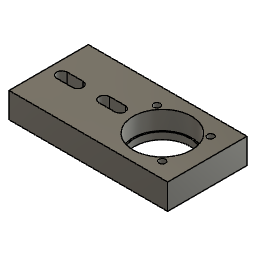
BeltTensionerBlock v21 (Autodesk Fusion 360 archive; units mm, degrees)
design "BeltTensionerBlock" references "tormach 770mx"
Autodesk Fusion 360 part; units mm, degrees
sketch "Sketch1" plane through (0, 0, 0) normal (0, 1, 0) x (1, 0, 0)
  line L0 (0, 0) -> (60, 0)
  line L1 (60, 0) -> (60, -30)
  line L2 (60, -30) -> (0, -30)
  line L3 (0, -30) -> (0, 0)
  line L4 (0, -15) -> (60, -15) construction
  line L5 (8, 0) -> (8, -30) construction
  line L6 (24, 0) -> (24, -30) construction
  line L7 (11, -13) -> (5, -13)
  arc A0 (5, -13) -> (5, -17) centre (5, -15) ccw
  line L8 (5, -17) -> (11, -17)
  arc A1 (11, -17) -> (11, -13) centre (11, -15) ccw
  line L9 (11, -15) -> (5, -15) construction
  line L10 (21, -17) -> (27, -17)
  arc A2 (27, -17) -> (27, -13) centre (27, -15) ccw
  line L11 (27, -13) -> (21, -13)
  arc A3 (21, -13) -> (21, -17) centre (21, -15) ccw
  line L12 (21, -15) -> (27, -15) construction
  line L13 (43, 0) -> (43, -30) construction
  point P0 (11, -15)
  point P1 (5, -15)
  point P2 (21, -15)
  point P3 (27, -15)
  dimension "d1" = 60
  dimension "d2" = 30
  dimension "d3" = 8
  dimension "d4" = 16
  dimension "d5" = 3
  dimension "d6" = 3
  dimension "d7" = 3
  dimension "d8" = 3
  dimension "d9" = 4
  dimension "d10" = 4
  dimension "d13" = 43
  constraint horizontal L0
  constraint vertical L1
  constraint horizontal L2
  constraint vertical L3
  constraint coincident L0.start L3.end
  constraint midpoint L3 L4.start
  constraint midpoint L1 L4.end
  constraint coincident L0 L5.start
  constraint coincident L2 L5.end
  constraint perpendicular L2 L5
  constraint coincident L0 L6.start
  constraint coincident L2 L6.end
  constraint perpendicular L2 L6
  constraint coincident L4 P0
  constraint coincident L4 P1
  constraint coincident L4 P2
  constraint coincident L4 P3
  constraint tangent L7 A0
  constraint tangent A0 L8
  constraint parallel L7 L8
  constraint tangent L8 A1
  constraint tangent L7 A1
  constraint coincident P1 A0.centre
  constraint perpendicular L5 L9
  constraint coincident P0 A1.centre
  constraint tangent L10 A2
  constraint tangent A2 L11
  constraint parallel L10 L11
  constraint tangent L11 A3
  constraint tangent L10 A3
  constraint coincident P3 A2.centre
  constraint perpendicular L6 L12
  constraint coincident P2 A3.centre
  constraint coincident L0 L13.start
  constraint coincident L2 L13.end
  constraint perpendicular L2 L13
  measures "d1" distance of L0.start L0.end
  measures "d2" distance of L0.start L2.end
  measures "d3" distance of L3 L5
  measures "d4" distance of L5 L6
  measures "d5" distance of L5 P1
  measures "d6" distance of L5 P0
  measures "d7" distance of L6 P2
  measures "d8" distance of L6 P3
  measures "d9" diameter of A0
  measures "d10" diameter of A2
  measures "d13" distance of L3 L13
extrude "Extrude1" add sketch "Sketch1" along normal blind 9.6
sketch "Sketch2" plane through (0, 9.6, 0) normal (0, 1, 0) x (-1, 0, 0)
  arc A0 (-21, 13) -> (-21, 17) centre (-21, 15) ccw
  line L0 (-21, 13) -> (-27, 13)
  arc A1 (-27, 17) -> (-27, 13) centre (-27, 15) ccw
  line L1 (-27, 17) -> (-21, 17)
  arc A2 (-11, 17) -> (-11, 13) centre (-11, 15) ccw
  line L2 (-11, 17) -> (-5, 17)
  arc A3 (-5, 13) -> (-5, 17) centre (-5, 15) ccw
  line L3 (-5, 13) -> (-11, 13)
  line L4 (0, 30) -> (-60, 30)
  line L5 (-60, 30) -> (-60, 0)
  line L6 (-60, 0) -> (0, 0)
  line L7 (0, 0) -> (0, 30)
  circle A4 centre (-43, 15) radius 11.05
  circle A5 centre (-43, 15) radius 10.55
  dimension "d15" = 22.1
  dimension "d16" = 21.1
  constraint concentric A4 A5
  measures "d15" diameter of A4
  measures "d16" diameter of A5
extrude "Extrude2" cut sketch "Sketch2" against normal blind 7 contours A4
extrude "Extrude3" cut 1 faces at (40.0944, 9.6, 14.0673) along direction (0, 1, 0) through all and the other way through all
sketch "Sketch3" plane through (0, 9.6, 0) normal (0, 1, 0) x (-1, 0, 0)
  line L0 (0, 30) -> (-60, 30)
  line L1 (-60, 30) -> (-60, 0)
  line L2 (-60, 0) -> (0, 0)
  line L3 (0, 0) -> (0, 30)
  arc A0 (-21, 13) -> (-21, 17) centre (-21, 15) ccw
  line L4 (-21, 13) -> (-27, 13)
  arc A1 (-27, 17) -> (-27, 13) centre (-27, 15) ccw
  line L5 (-27, 17) -> (-21, 17)
  arc A2 (-11, 17) -> (-11, 13) centre (-11, 15) ccw
  line L6 (-11, 17) -> (-5, 17)
  arc A3 (-5, 13) -> (-5, 17) centre (-5, 15) ccw
  line L7 (-5, 13) -> (-11, 13)
  circle A4 centre (-43, 15) radius 11.05
  circle A5 centre (-43, 15) radius 13 construction
  point P0 (-32.8444, 6.8844)
  point P1 (-52.1828, 24.202)
  point P2 (-53.1556, 6.8844)
  dimension "d30" = 26
  constraint concentric A4 A5
  constraint coincident A5 P0
  constraint coincident A5 P1
  constraint coincident A5 P2
  measures "d30" diameter of A5
hole "Hole1" at (32.8444, 9.6, 6.8844) direction (0, -1, 0) diameter 2.5 end through all
hole "Hole2" at (53.1556, 9.6, 6.8844) direction (0, -1, 0) diameter 2.5 end through all
hole "Hole3" at (52.1828, 9.6, 24.202) direction (0, -1, 0) diameter 2.5 end through all
